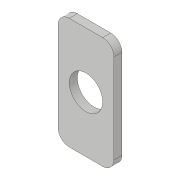
# Autodesk Inventor part: 20_Cube_Insert_Sample_clamp
Saved by Autodesk Inventor 2022 (Build 260153000, 153)
## iProperties
Created: 2019-08-09
Part Number: 20_Cube_Insert_Sample_clamp
Material: Generic
Document SubType Name: Modeling
Designer: marsikovabarbora
Density: 1 g/cm^3
Appearance: Default
Catalog Web Link: isPrinted
Vendor: openUC2
Author: marsikovabarbora
Autodesk Inventor part; units mm, degrees
ref_plane "YZ Plane" through (0, 0, 0) normal (1, 0, 0) x (0, 1, 0)
ref_plane "XZ Plane" through (0, 0, 0) normal (0, 1, 0) x (-1, 0, 0)
ref_plane "XY Plane" through (0, 0, 0) normal (0, 0, 1) x (1, 0, 0)
sketch "Sketch1" plane through (0, 0, 0) normal (0, 0, 1) x (1, 0, 0)
  line L0 (0, -36.3851) -> (0, 36.5144) construction
  circle A0 centre (0, 0.0647) radius 20
  circle A1 centre (0, 20.0647) radius 4.05
  circle A2 centre (0, -19.9353) radius 4.05
  line L1 (7.5, -24.9353) -> (-7.5, -24.9353)
  line L2 (-12.5, -19.9353) -> (-12.5, 20.0647)
  line L3 (-7.5, 25.0647) -> (7.5, 25.0647)
  line L4 (12.5, 20.0647) -> (12.5, -19.9353)
  line L5 (12.5, -24.9353) -> (-12.5, 25.0647) construction
  line L6 (-12.5, -24.9353) -> (12.5, 25.0647) construction
  arc A3 (-7.5, 25.0647) -> (-12.5, 20.0647) centre (-7.5, 20.0647) ccw
  arc A4 (12.5, 20.0647) -> (7.5, 25.0647) centre (7.5, 20.0647) ccw
  arc A5 (7.5, -24.9353) -> (12.5, -19.9353) centre (7.5, -19.9353) ccw
  arc A6 (-12.5, -19.9353) -> (-7.5, -24.9353) centre (-7.5, -19.9353) ccw
  circle A7 centre (0, 0.0647) radius 7.5
  dimension "d6" = 40
  dimension "d7" = 8.1
  dimension "d8" = 8.1
  dimension "d9" = 25
  dimension "d10" = 50
  dimension "d11" = 5
  dimension "d12" = 15
  constraints: 12 end point, 10 point on circle, 10 point on line, 8 centre point, 8 tangent, 3 equal radius, 3 midpoint, 2 parallel, 1 coincident, 1 horizontal, 1 perpendicular
  measures "d6" diameter of A0
  measures "d7" diameter of A1
  measures "d8" diameter of A2
  measures "d9" distance of L5.end L6.end
  measures "d10" distance of L6.start L5.end
  measures "d11" radius of A3
  measures "d12" diameter of A7
extrude "Extrusion1" add sketch "Sketch1" along normal blind 3 contours L4 A0 A2 L2 A1 | A0 A1 L2 A3 L3 A4 L4 | L4 A5 L1 A6 L2 A0 A2
sketch "Skizze2" plane through (0, 0, 3) normal (0, 0, 1) x (1, 0, 0)
  circle A0 centre (0, 20.0647) radius 4.05 projected
  circle A1 centre (0, 0.0647) radius 7.5 projected
  circle A2 centre (0, -19.9353) radius 4.05 projected
  arc A3 (12.5, 20.0647) -> (7.5, 25.0647) centre (7.5, 20.0647) ccw projected
  line L0 (7.5, 25.0647) -> (-7.5, 25.0647) projected
  arc A4 (-7.5, 25.0647) -> (-12.5, 20.0647) centre (-7.5, 20.0647) ccw projected
  line L1 (-12.5, 20.0647) -> (-12.5, -19.9353) projected
  arc A5 (-12.5, -19.9353) -> (-7.5, -24.9353) centre (-7.5, -19.9353) ccw projected
  line L2 (-7.5, -24.9353) -> (7.5, -24.9353) projected
  arc A6 (7.5, -24.9353) -> (12.5, -19.9353) centre (7.5, -19.9353) ccw projected
  line L3 (12.5, -19.9353) -> (12.5, 20.0647) projected
  point P0 (0, 0)
extrude "Extrusion2" add sketch "Skizze2" along normal blind 0.6 contours A0 | A2 | L3 A6 L2 A5 L1 A4 L0 A3
body "Solid1"
